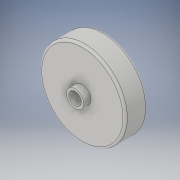
# Autodesk Inventor part: Bauteil1
Saved by Autodesk Inventor 2019 (Build 230136000, 136)
## iProperties
Created: 2024-05-17
Part Number: Bauteil1
Material: Generisch
Document SubType Name: Modeling
Designer: nic
Density: 1 g/cm^3
Appearance: Vorgabe
Author: nic
Autodesk Inventor part; units mm, degrees
ref_plane "YZ Plane" through (0, 0, 0) normal (1, 0, 0) x (0, 1, 0)
ref_plane "XZ Plane" through (0, 0, 0) normal (0, 1, 0) x (-1, 0, 0)
ref_plane "XY Plane" through (0, 0, 0) normal (0, 0, 1) x (1, 0, 0)
sketch "Skizze1" plane through (0, 0, 0) normal (0, 0, 1) x (1, 0, 0)
  circle A0 centre (0, 0) radius 77
  circle A1 centre (0, 0) radius 11.415
  dimension "d0" = 154
  dimension "d1" = 22.83
  constraints: 2 centre point, 2 coincident
  measures "d0" diameter of A0
  measures "d1" diameter of A1
extrude "Extrusion1" add sketch "Skizze1" along normal blind 40.6
sketch "Skizze2" plane through (0, 0, 0) normal (0, 0, -1) x (-1, 0, 0)
  circle A0 centre (0, 0) radius 16.25
  dimension "d4" = 32.5
  constraints: 1 centre point, 1 coincident
  measures "d4" diameter of A0
extrude "Extrusion2" cut sketch "Skizze2" against normal blind 11
sketch "Skizze3" plane through (0, 0, 11) normal (0, 0, -1) x (-1, 0, 0)
  circle A0 centre (0, 0) radius 15
  dimension "d7" = 30
  constraints: 1 centre point, 1 coincident
  measures "d7" diameter of A0
extrude "Extrusion3" cut sketch "Skizze3" against normal blind 8
fillet "Rundung1" radius 2 1 edges at (15, 0, 11)
fillet "Rundung2" radius 2 1 edges at (16.25, 0, 0)
fillet "Rundung3" radius 4 2 edges at (-77, 0, 0) (-77, 0, 40.6)
sketch "Skizze4" plane through (0, 0, 40.6) normal (0, 0, 1) x (1, 0, 0)
  circle A0 centre (0, 0) radius 11.415 projected
  circle A1 centre (0, 0) radius 15.415
  dimension "d13" = 4
  constraints: 1 centre point
  measures "d13" radial gap between concentric circles of A0 A1
extrude "Extrusion4" add sketch "Skizze4" along normal blind 13
